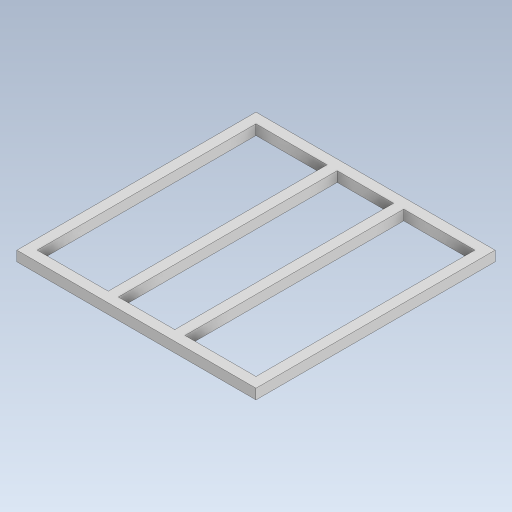
# Autodesk Inventor part: MockChassis(delete asap)
Saved by Autodesk Inventor 2023 (Build 270158000, 158)
## iProperties
Created: 2023-04-10
Part Number: MockChassis(delete asap)
Material: Generic
Document SubType Name: Modeling
Designer: Dave
Density: 1 g/cm^3
Appearance: Default
Author: Dave
Autodesk Inventor part; units mm, degrees
ref_plane "YZ Plane" through (0, 0, 0) normal (1, 0, 0) x (0, 1, 0)
ref_plane "XZ Plane" through (0, 0, 0) normal (0, 1, 0) x (-1, 0, 0)
ref_plane "XY Plane" through (0, 0, 0) normal (0, 0, 1) x (1, 0, 0)
sketch "Sketch1" plane through (0, 0, 0) normal (0, 1, 0) x (-1, 0, 0)
  line L0 (300, 300) -> (-300, 300)
  line L1 (-300, 300) -> (-300, -300)
  line L2 (-300, -300) -> (300, -300)
  line L3 (300, -300) -> (300, 300)
  line L4 (300, 300) -> (-300, -300) construction
  line L5 (-300, 300) -> (300, -300) construction
  line L6 (274.6, 274.6) -> (-274.6, 274.6)
  line L7 (-274.6, 274.6) -> (-274.6, -274.6)
  line L8 (-274.6, -274.6) -> (274.6, -274.6)
  line L9 (274.6, -274.6) -> (274.6, 274.6)
  line L10 (-70.84, -274.6) -> (-70.84, 274.6)
  line L11 (-96.24, 274.6) -> (-96.24, -274.6)
  line L12 (96.24, -274.6) -> (96.24, 274.6)
  line L13 (70.84, 274.6) -> (70.84, -274.6)
  line L14 (0, 0) -> (0, -274.6) construction
  dimension "d0" = 600
  dimension "d1" = 600
  dimension "d2" = 25.4
  dimension "d3" = 25.4
  dimension "d4" = 396.24
  constraints: 30 end point, 8 point on line, 6 perpendicular, 4 parallel, 3 midpoint, 1 horizontal, 5 other
  measures "d0" distance of L2.end L1.end
  measures "d1" distance of L1.end L0.end
  measures "d2" distance between parallel lines of L3 L9
  measures "d3" distance between parallel lines of L12 L13
  measures "d4" distance between parallel lines of L11 L3
extrude "Extrusion1" add sketch "Sketch1" along normal blind 25.4 contours L3 L2 L1 L0 | L12 L8 L13 L6 | L10 L8 L11 L6
body "Solid1"
